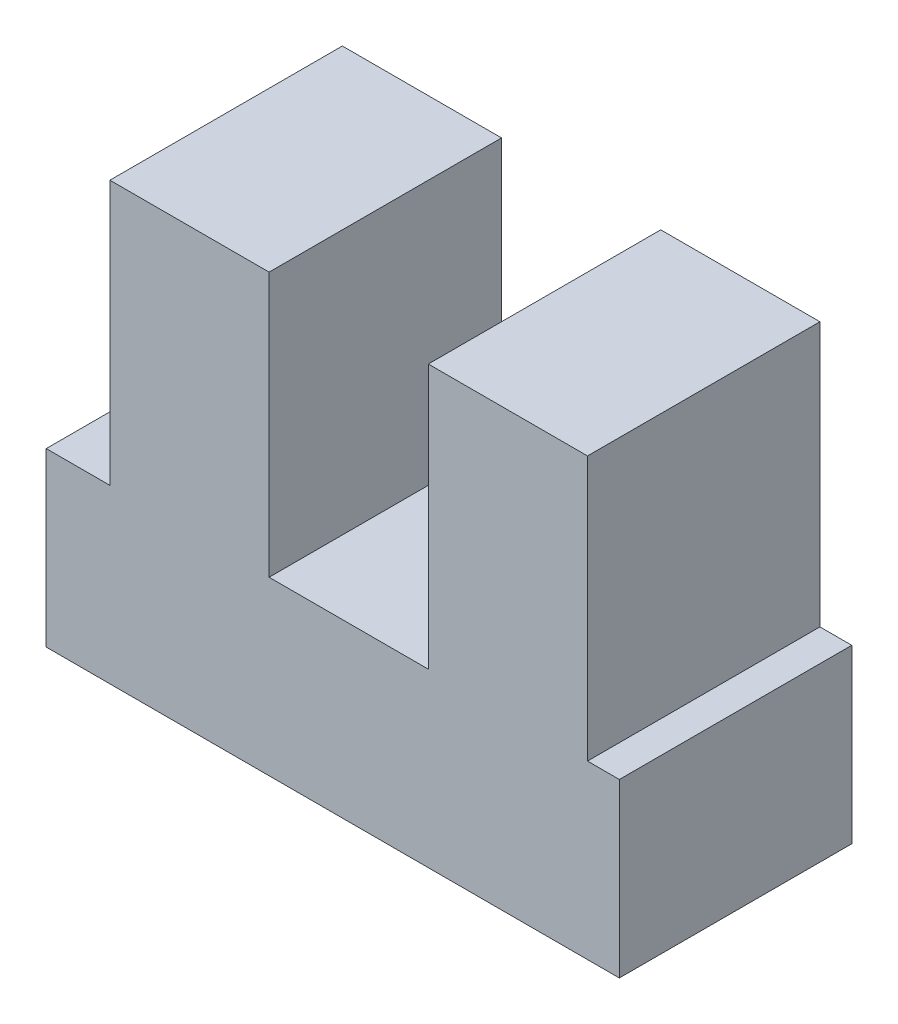
# Autodesk Inventor part: Part2
Saved by Autodesk Inventor 2019 (Build 230136000, 136)
## iProperties
Created: 2018-11-27
Part Number: Part2
Material: Generic
Document SubType Name: Modeling
Designer: Andres
Density: 1 g/cm^3
Appearance: Default
Author: Andres
Autodesk Inventor part; units mm, degrees
ref_plane "YZ Plane" through (0, 0, 0) normal (1, 0, 0) x (0, 1, 0)
ref_plane "XZ Plane" through (0, 0, 0) normal (0, 1, 0) x (-1, 0, 0)
ref_plane "XY Plane" through (0, 0, 0) normal (0, 0, 1) x (1, 0, 0)
sketch "Sketch1" plane through (0, 0, 0) normal (0, 0, 1) x (1, 0, 0)
  line L0 (-9, 2.7) -> (9, 2.7)
  line L1 (9, 2.7) -> (9, -2.7)
  line L2 (9, -2.7) -> (-9, -2.7)
  line L3 (-9, -2.7) -> (-9, 2.7)
  line L4 (-9, 2.7) -> (9, -2.7) construction
  line L5 (9, 2.7) -> (-9, -2.7) construction
  line L6 (3, 11) -> (8, 11)
  line L7 (8, 11) -> (8, 2.7)
  line L8 (8, 2.7) -> (3, 2.7)
  line L9 (3, 2.7) -> (3, 11)
  line L10 (3, 11) -> (8, 2.7) construction
  line L11 (8, 11) -> (3, 2.7) construction
  line L12 (-7, 11) -> (-2, 11)
  line L13 (-2, 11) -> (-2, 2.7)
  line L14 (-2, 2.7) -> (-7, 2.7)
  line L15 (-7, 2.7) -> (-7, 11)
  line L16 (-7, 11) -> (-2, 2.7) construction
  line L17 (-2, 11) -> (-7, 2.7) construction
  point P0 (0, 0)
  point P1 (5.5, 6.85)
  point P2 (-4.5, 6.85)
  dimension "d0" = 18
  dimension "d1" = 5.4
  dimension "d2" = 5
  dimension "d3" = 8.3
  dimension "d4" = 1
  dimension "d5" = 5
  dimension "d6" = 8.3
  dimension "d7" = 5
  constraints: 36 end point, 6 midpoint, 6 parallel, 3 horizontal, 3 perpendicular, 2 point on line
  measures "d0" distance of L1.end L2.end
  measures "d1" distance of L0.end L1.end
  measures "d2" distance of L7.end L8.end
  measures "d3" distance of L6.end L7.end
  measures "d4" distance between parallel lines of L1 L7
  measures "d5" distance of L13.end L14.end
  measures "d6" distance of L12.end L13.end
  measures "d7" distance between parallel lines of L9 L13
extrude "Extrusion1" add sketch "Sketch1" along normal blind 7.3
body "Solid1"
